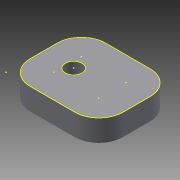
# Autodesk Inventor part: Pseudo-Guitar
Saved by Autodesk Inventor 2014 SP1 (Build 180222100, 222)
## iProperties
Created: 2016-11-27
Part Number: Pseudo-Guitar
Material: Generic
Document SubType Name: Modeling
Designer: danielsikar
Density: 1 g/cm^3
Appearance: Default
Author: danielsikar
Autodesk Inventor part; units mm, degrees
ref_plane "YZ Plane" through (0, 0, 0) normal (1, 0, 0) x (0, 1, 0)
ref_plane "XZ Plane" through (0, 0, 0) normal (0, 1, 0) x (-1, 0, 0)
ref_plane "XY Plane" through (0, 0, 0) normal (0, 0, 1) x (1, 0, 0)
sketch "Sketch1" plane through (0, 0, 0) normal (0, 0, 1) x (1, 0, 0)
  line L0 (0, 0) -> (465, 0)
  line L1 (465, 0) -> (465, 377)
  line L2 (465, 377) -> (0, 377)
  line L3 (0, 377) -> (0, 0)
  line L4 (0, 188.5) -> (465, 188.5) construction
  line L5 (150, 478.4047) -> (150, -123.5436) construction
  circle A0 centre (150, 188.5) radius 42.3
  dimension "d0" = 465
  dimension "d1" = 377
  dimension "d7" = 315
  dimension "d8" = 84.6
  constraints: 12 end point, 2 midpoint, 2 parallel, 2 perpendicular, 2 point on line, 1 centre point, 1 horizontal
  measures "d0" distance of L2.end L1.end
  measures "d1" distance of L1.end L0.end
  measures "d7" distance between parallel lines of L5 L1
  measures "d8" diameter of A0
extrude "Extrusion1" add sketch "Sketch1" along normal blind 3
sketch "Sketch2" plane through (0, 0, 0) normal (0, 0, -1) x (-1, 0, 0)
  circle A0 centre (-150, 188.5) radius 42.3 projected
  line L0 (-465, 377) -> (0, 377)
  line L1 (0, 377) -> (0, 0)
  line L2 (0, 0) -> (-465, 0)
  line L3 (-465, 0) -> (-465, 377)
  constraints: 8 end point, 2 parallel, 1 horizontal, 1 perpendicular
extrude "Extrusion2" add sketch "Sketch2" along normal blind 106
sketch "Sketch3" plane through (0, 0, -106) normal (0, 0, -1) x (-1, 0, 0)
  circle A0 centre (-150, 188.5) radius 42.3 projected
  circle A1 centre (-150, 188.5) radius 50.9763
  constraints: 1 centre point, 1 coincident
extrude "Extrusion3" add sketch "Sketch3" against normal blind 10.9 contours A0
fillet "Fillet1" radius 120 4 edges at (465, 0, -51.5) (465, 377, -51.5) (0, 0, -51.5) (0, 377, -51.5)
sketch "Sketch4" plane through (0, 0, 3) normal (0, 0, 1) x (1, 0, 0)
  arc A0 (120, 377) -> (0, 257) centre (120, 257) ccw projected
  line L0 (0, 257) -> (0, 120) projected
  arc A1 (0, 120) -> (120, 0) centre (120, 120) ccw projected
  line L1 (120, 0) -> (345, 0) projected
  arc A2 (345, 0) -> (465, 120) centre (345, 120) ccw projected
  line L2 (465, 120) -> (465, 257) projected
  arc A3 (465, 257) -> (345, 377) centre (345, 257) ccw projected
  line L3 (345, 377) -> (120, 377) projected
  circle A4 centre (150, 188.5) radius 42.3 projected
  point P0 (0, 0)
shell "Shell1" thickness 3 removed faces 1 at (195, 125.6667, -106)
body "Solid1"
